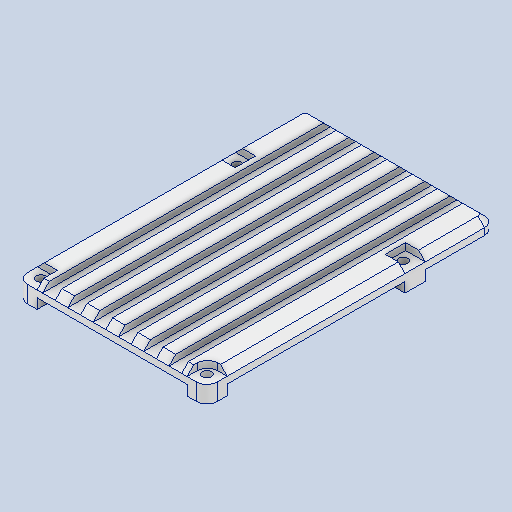
# Autodesk Inventor part: Raspberry-Pi-4B heatsink1
Saved by Autodesk Inventor 2023 (Build 270158000, 158)
## iProperties
Created: 2023-04-10
Part Number: Raspberry-Pi-4B heatsink1
Material: Aluminum 6061
Document SubType Name: Modeling
Designer: ASARe-DAQ-PC
Density: 2.7 g/cm^3
Appearance: Aluminum - Flat
Mass: 39.9563 g
Surface Area: 126.894 cm^2
Volume: 14.7986 cm^3
Author: ASARe-DAQ-PC
Autodesk Inventor part; units mm, degrees
ref_plane "YZ Plane" through (0, 0, 0) normal (1, 0, 0) x (0, 1, 0)
ref_plane "XZ Plane" through (0, 0, 0) normal (0, 1, 0) x (-1, 0, 0)
ref_plane "XY Plane" through (0, 0, 0) normal (0, 0, 1) x (1, 0, 0)
sketch "Sketch1" plane through (0, 0, 0) normal (0, 1, 0) x (-1, 0, 0)
  line L0 (3, 0) -> (53, 0)
  line L1 (56, -3) -> (56, -82)
  line L2 (53, -85) -> (3, -85)
  line L3 (0, -82) -> (0, -3)
  arc A0 (56, -3) -> (53, 0) centre (53, -3) ccw
  arc A1 (53, -85) -> (56, -82) centre (53, -82) ccw
  arc A2 (0, -82) -> (3, -85) centre (3, -82) ccw
  arc A3 (3, 0) -> (0, -3) centre (3, -3) ccw
  point P0 (0, 0)
  point P1 (56, 0)
  point P2 (0, -85)
  dimension "d0" = 56
  dimension "d1" = 85
  dimension "d2" = 3
  constraints: 8 end point, 8 point on circle, 8 tangent, 6 point on line, 4 centre point, 3 equal radius, 2 parallel, 1 horizontal, 1 perpendicular
  measures "d0" distance of point (0, 0) point (56, 0)
  measures "d1" distance of point (0, -85) point (0, 0)
  measures "d2" radius of A0
extrude "Extrusion1" add sketch "Sketch1" along normal blind 4
chamfer "Chamfer1" distance 2 angle 45 8 edges at (0, 4, -42.5) (-0.8787, 4, -84.1213) (-28, 4, -85) (-55.1213, 4, -84.1213) (-56, 4, -42.5) (-55.1213, 4, -0.8787) (-28, 4, 0) (-0.8787, 4, -0.8787)
sketch "Sketch2" plane through (0, 0, 0) normal (0, 1, 0) x (-1, 0, 0)
  line L0 (53, 0) -> (3, 0) projected
  line L1 (3, -85) -> (53, -85) projected
  line L2 (44.8, 0) -> (48.5333, 0)
  line L3 (48.5333, 0) -> (48.5333, -85)
  line L4 (48.5333, -85) -> (44.8, -85)
  line L5 (44.8, -85) -> (44.8, 0)
  line L6 (56, -82) -> (56, -3) projected
  line L7 (41.0667, 0) -> (44.8, 0)
  line L8 (44.8, 0) -> (44.8, -85)
  line L9 (44.8, -85) -> (41.0667, -85)
  line L10 (41.0667, -85) -> (41.0667, 0)
  line L11 (37.3334, 0) -> (41.0667, 0)
  line L12 (41.0667, 0) -> (41.0667, -85)
  line L13 (41.0667, -85) -> (37.3334, -85)
  line L14 (37.3334, -85) -> (37.3334, 0)
  line L15 (33.6001, 0) -> (37.3334, 0)
  line L16 (37.3334, 0) -> (37.3334, -85)
  line L17 (37.3334, -85) -> (33.6001, -85)
  line L18 (33.6001, -85) -> (33.6001, 0)
  line L19 (29.8668, 0) -> (33.6001, 0)
  line L20 (33.6001, 0) -> (33.6001, -85)
  line L21 (33.6001, -85) -> (29.8668, -85)
  line L22 (29.8668, -85) -> (29.8668, 0)
  line L23 (26.1335, 0) -> (29.8668, 0)
  line L24 (29.8668, 0) -> (29.8668, -85)
  line L25 (29.8668, -85) -> (26.1335, -85)
  line L26 (26.1335, -85) -> (26.1335, 0)
  line L27 (22.4002, 0) -> (26.1335, 0)
  line L28 (26.1335, 0) -> (26.1335, -85)
  line L29 (26.1335, -85) -> (22.4002, -85)
  line L30 (22.4002, -85) -> (22.4002, 0)
  line L31 (18.6669, 0) -> (22.4002, 0)
  line L32 (22.4002, 0) -> (22.4002, -85)
  line L33 (22.4002, -85) -> (18.6669, -85)
  line L34 (18.6669, -85) -> (18.6669, 0)
  line L35 (14.9336, 0) -> (18.6669, 0)
  line L36 (18.6669, 0) -> (18.6669, -85)
  line L37 (18.6669, -85) -> (14.9336, -85)
  line L38 (14.9336, -85) -> (14.9336, 0)
  line L39 (11.2003, 0) -> (14.9336, 0)
  line L40 (14.9336, 0) -> (14.9336, -85)
  line L41 (14.9336, -85) -> (11.2003, -85)
  line L42 (11.2003, -85) -> (11.2003, 0)
  line L43 (7.467, 0) -> (11.2003, 0)
  line L44 (11.2003, 0) -> (11.2003, -85)
  line L45 (11.2003, -85) -> (7.467, -85)
  line L46 (7.467, -85) -> (7.467, 0)
  point P0 (0, 0)
  dimension "d8" = 7.4667
  dimension "d9" = 3.7333
  dimension "d12" = 3.7333
  constraints: 88 end point, 2 horizontal, 2 parallel, 2 point on line, 1 perpendicular, 80 other
  measures "d8" distance between parallel lines of L6 L3
  measures "d9" distance between parallel lines of L5 L3
  measures "d12" distance of L2.start L7.start
extrude "Extrusion2" cut sketch "Sketch2" against normal blind 2 from surface at 4 contours L3 L1 L5 L0 | L10 L1 L14 L0 | L18 L1 L22 L0 | L26 L1 L30 L0 | L34 L1 L38 L0 | L42 L1 L46 L0
sketch "Sketch3" plane through (0, 0, 0) normal (0, -1, 0) x (1, 0, 0)
  line L0 (-3, 0) -> (-5.85, 0)
  line L1 (-5.85, 0) -> (-5.85, -3)
  line L2 (-2.85, -6) -> (0, -6)
  line L3 (0, -6) -> (0, -3)
  line L4 (0, -3) -> (0, -82) projected
  line L5 (0, -58.5) -> (-4.467, -58.5)
  line L6 (-5.85, -64.5) -> (-5.85, -64.5)
  line L7 (-4.467, -64.5) -> (0, -64.5)
  line L8 (0, -64.5) -> (0, -58.5)
  line L9 (-28, 0) -> (-28, -85) construction
  line L10 (-53, 0) -> (-3, 0) projected
  line L11 (-3, -85) -> (-53, -85) projected
  arc A0 (0, -3) -> (-3, 0) centre (-3, -3) ccw
  arc A1 (-5.85, -3) -> (-2.85, -6) centre (-2.85, -3) ccw
  line L12 (0, -6) -> (-5.85, -6)
  line L13 (0, -58.5) -> (-2.85, -58.5)
  line L14 (-2.85, -64.5) -> (0, -64.5)
  line L15 (-5.85, -61.5) -> (-5.85, -61.5)
  arc A2 (-2.85, -58.5) -> (-5.85, -61.5) centre (-2.85, -61.5) ccw
  arc A3 (-5.85, -61.5) -> (-2.85, -64.5) centre (-2.85, -61.5) ccw
  line L16 (0, -58.5) -> (-5.85, -58.5)
  line L17 (-5.85, -58.5) -> (-5.85, -64.5)
  line L18 (-5.85, -64.5) -> (0, -64.5)
  line L19 (0, -3) -> (0, -82) projected
  line L20 (-5.85, -6) -> (-5.85, 0)
  line L21 (-53, 0) -> (-50.15, 0)
  line L22 (-50.15, 0) -> (-50.15, -3)
  line L23 (-53.15, -6) -> (-56, -6)
  line L24 (-56, -6) -> (-56, -3)
  line L25 (-56, -58.5) -> (-51.533, -58.5)
  line L26 (-50.15, -64.5) -> (-50.15, -64.5)
  line L27 (-51.533, -64.5) -> (-56, -64.5)
  line L28 (-56, -64.5) -> (-56, -58.5)
  arc A4 (-53, 0) -> (-56, -3) centre (-53, -3) ccw
  arc A5 (-53.15, -6) -> (-50.15, -3) centre (-53.15, -3) ccw
  line L29 (-56, -6) -> (-50.15, -6)
  line L30 (-56, -58.5) -> (-53.15, -58.5)
  line L31 (-53.15, -64.5) -> (-56, -64.5)
  line L32 (-50.15, -61.5) -> (-50.15, -61.5)
  arc A6 (-50.15, -61.5) -> (-53.15, -58.5) centre (-53.15, -61.5) ccw
  arc A7 (-53.15, -64.5) -> (-50.15, -61.5) centre (-53.15, -61.5) ccw
  line L33 (-56, -58.5) -> (-50.15, -58.5)
  line L34 (-50.15, -58.5) -> (-50.15, -64.5)
  line L35 (-50.15, -64.5) -> (-56, -64.5)
  line L36 (-50.15, -6) -> (-50.15, 0)
  point P0 (0, 0)
  point P1 (-7.467, 0)
  point P2 (-2.2335, -58.5)
  point P3 (0, -64.5)
  point P4 (-7.467, -2)
  point P5 (-56, 0)
  point P6 (-48.533, 0)
  point P7 (-56, -3)
  point P8 (-53.7665, -58.5)
  point P9 (-53, 0)
  point P10 (-48.533, -2)
  point P11 (-53.15, -58.5)
  point P12 (-5.85, -61.5)
  point P13 (-2.85, -64.5)
  point P14 (-2.85, -58.5)
  point P15 (-50.15, 0)
  point P16 (-2.85, -6)
  dimension "d19" = 6
  dimension "d21" = 58.5
  dimension "d22" = 6
  dimension "d25" = 28
  dimension "d26" = 3
  dimension "d29" = 3
  dimension "d30" = 3
  dimension "d48" = 5.85
  constraints: 66 end point, 29 symmetric about line, 25 point on line, 16 point on circle, 8 centre point, 8 tangent, 5 midpoint, 5 parallel, 3 perpendicular, 2 collinear, 2 horizontal, 1 concentric, 1 vertical, 4 other
  measures "d19" distance between parallel lines of L0 L2
  measures "d21" distance between parallel lines of L0 L5
  measures "d22" distance from line of point (-2.233, -58.5) L7
  measures "d25" distance between parallel lines of L4 L9
  measures "d26" radius of A0
  measures "d29" radius of A1
  measures "d30" radius of A2
  measures "d48" distance between parallel lines of L8 L17
extrude "Extrusion3" add sketch "Sketch3" along normal blind 3 contours A0 L3 L2 A1 L1 L0 | L4 L7 A3 A2 L5 | L22 A5 L23 L24 A4 L10 | L25 A6 A7 L27 L28
extrude "Extrusion4" cut sketch "Sketch3" along normal blind 2 from surface at -4 contours A0 L3 L2 A1 L1 L0 | L4 L7 A3 A2 L5 | L22 A5 L23 L24 A4 L10 | L36 L29 A5 | A2 L17 L16 L5 | L7 L18 L17 A3 | L25 A6 A7 L27 L28 | L25 L33 L34 A6 | L34 L35 L27 A7
sketch "Sketch4" plane through (-53, 2, 0) normal (0, 1, 0) x (1, 0, 0)
  line L0 (-0.15, 58.5) -> (-3, 58.5) projected
  line L1 (-3, 64.5) -> (-3, 58.5) projected
  line L2 (-3, 6) -> (-3, 3) projected
  line L3 (0, 0) -> (2.85, 0) projected
  line L4 (47.15, 0) -> (50, 0) projected
  line L5 (53, 3) -> (53, 6) projected
  line L6 (53, 58.5) -> (53, 64.5) projected
  line L7 (50.15, 64.5) -> (53, 64.5) projected
  point P0 (0.5, 3.5)
  point P1 (0.5, 61.5)
  point P2 (49.5, 61.5)
  point P3 (49.5, 3.5)
  dimension "d49" = 3
  dimension "d50" = 3.5
  dimension "d51" = 3.5
  dimension "d52" = 3.5
  dimension "d53" = 3.5
  dimension "d54" = 3.5
  dimension "d55" = 3.5
  dimension "d56" = 3
  measures "d49" distance from line of L0 point (0.5, 61.5)
  measures "d50" distance from line of point (0.5, 61.5) L1
  measures "d51" distance from line of L2 point (0.5, 3.5)
  measures "d52" distance from line of L3 point (0.5, 3.5)
  measures "d53" distance from line of L4 point (49.5, 3.5)
  measures "d54" distance from line of L5 point (49.5, 3.5)
  measures "d55" distance from line of L6 point (49.5, 61.5)
  measures "d56" distance from line of L7 point (49.5, 61.5)
hole "Hole1" at (-52.5, 2, -3.5) at (-52.5, 2, -61.5) at (-3.5, 2, -61.5) at (-3.5, 2, -3.5) direction (0, -1, 0) diameter 2.7 end through all
body "Solid1"
